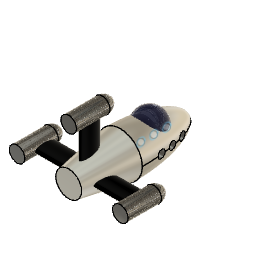
P2 (Autodesk Fusion 360 design; units mm, degrees)
Autodesk Fusion 360 part; units mm, degrees
sketch "Sketch1" plane through (0, 0, 0) normal (0, 1, 0) x (1, 0, 0)
  circle A0 centre (0, 0) radius 25
  dimension "d1" = 50
  constraint coincident A0.centre origin
  measures "d1" diameter of A0
extrude "Extrude1" add sketch "Sketch1" along normal blind 100 draft 10 makes body 1
sketch "Sketch2" plane through (0, 0, 0) normal (0, 0, 1) x (1, 0, 0)
  line L0 (0, 100) -> (42.5, 100)
  line L1 (0, 100) -> (0, 105)
  line L2 (0, 105) -> (0, 230)
  ellipse E0 centre (0, 100) end of major axis (0, 230) minor radius 42.5 (42.5, 100) -> (0, 230) ccw
  dimension "d6" = 42.5
  dimension "d7" = 125
  constraint horizontal L0
  constraint perpendicular L0 L1
  constraint perpendicular L0 L2
  constraint coincident L0.start L1.start
  measures "d6" distance of L0.start L0.end
  measures "d7" distance of L1.end L2.end
revolve "Revolve1" add sketch "Sketch2" angle 360 about axis through (0, 105, 0) along (0, 1, 0) separate body makes body 2
sketch "Sketch3" plane through (0, 0, 0) normal (0, 0, 1) x (1, 0, 0)
  line L0 (0, 0) -> (0, 20)
  line L1 (0, 40) -> (0, 60)
  ellipse E0 centre (0, 40) end of major axis (0, 60) minor radius 7
  line L2 (0, 20) -> (0, 60) construction
  line L3 (7, 40) -> (-7, 40) construction
  dimension "d9" = 20
  dimension "d10" = 7
  constraint coincident L0.start origin
  constraint vertical L0
  constraint parallel L0 L1
  constraint coincident E0 L0.end
  constraint coincident E0 L1.end
  constraint coincident E0 L3.start
  constraint coincident E0 L3.end
  constraint coincident L1.start E0.centre
  constraint coincident L1.end L2.end
  measures "d9" distance of L1.start L1.end
  measures "d10" distance of L1.start L3.start
extrude "Extrude2" add sketch "Sketch3" along normal blind 100 separate body makes body 3
sketch "Sketch6" plane through (0, 0, 100) normal (0, 0, 1) x (-1, 0, 0)
  ellipse E0 centre (0, -40) end of major axis (0, -60) minor radius 7
sketch "Sketch7" plane through (0, 0, 0) normal (0, 0, 1) x (1, 0, 0)
sketch "Sketch8" plane through (0, 0, 100) normal (0, 0, 1) x (1, 0, 0)
  line L0 (0, 0) -> (0, 65)
  line L1 (15, 65) -> (15, 0)
  line L2 (15, 0) -> (0, 0)
  line L3 (0, 65) -> (0, 66.0302)
  line L4 (0, 66.0302) -> (0, 84.3649)
  arc A0 (15, 65) -> (0, 84.3649) centre (-5, 65) ccw
  dimension "d16" = 65
  dimension "d17" = 5
  dimension "d18" = 40
  constraint coincident L0.start L2.end
  constraint vertical L0
  constraint tangent L1 A0
  constraint vertical L1
  constraint perpendicular L0 L2
  measures "d16" distance of L0.start L0.end
  measures "d17" distance of L0.end A0.centre
  measures "d18" diameter of A0
revolve "Revolve2" add sketch "Sketch8" angle 360 about axis through (0, 0, 100) along (0, 1, 0) separate body makes body 4
pattern_circular "C-Pattern1" count 3 over 180 about axis through (0, 1.75, 0) along (0, 1, 0) both ways of bodies 3 4 makes body 5 at (-66.6667, 40.8244, 6.9941) makes body 6 at (66.6667, 40.8244, -6.9941) makes body 7 at (-100.7477, 43.3333, 14.9814) makes body 8 at (100.7477, 43.3333, -14.9814)
sketch "Sketch9" plane through (0, 0, 100) normal (0, 0, 1) x (1, 0, 0)
sketch "Sketch10" plane through (0, 0, 0) normal (1, 0, 0) x (0, 1, 0)
  circle A0 centre (140, 0) radius 7.5
  circle A1 centre (165, 0) radius 7.5
  circle A2 centre (190, 0) radius 7.5
  dimension "d25" = 25
  dimension "d26" = 25
  dimension "d27" = 15
  dimension "d28" = 15
  dimension "d29" = 15
  measures "d25" distance of A1.centre A2.centre
  measures "d26" distance of A0.centre A1.centre
  measures "d27" diameter of A0
  measures "d28" diameter of A1
  measures "d29" diameter of A2
extrude "Extrude4" cut sketch "Sketch10" against normal blind 25 from surface at 42.5 bodies 2
pattern_circular "C-Pattern2" count 2 over 360 about axis through (0, 1.75, 0) along (0, 1, 0) of "Extrude4"
sketch "Sketch11" plane through (0, 0, 0) normal (1, 0, 0) x (0, 1, 0)
  line L0 (0, 35) -> (1.6504, 35)
  arc A0 (183.4345, 4.6946) -> (131.6504, 35) centre (157.5424, 19.8473) ccw
  line L1 (183.4345, 4.6946) -> (131.6504, 35)
  dimension "d37" = 35
  dimension "d40" = 130
  dimension "d41" = 30
  measures "d37" distance of origin L0.start
  measures "d40" distance of L0.end A0.end
  measures "d41" distance of A0.end A0.centre
revolve "Revolve3" add sketch "Sketch11" angle 360 about axis through (0, 183.4345, 4.6946) along (0, -0.863067, 0.50509) separate body makes body 9
